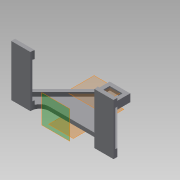
# Autodesk Inventor part: 11_Objektaufnahme
Saved by Autodesk Inventor 2015 (Build 190159000, 159)
## iProperties
Created: 2015-10-26
Part Number: 11_Objektaufnahme
Material: Generisch
Document SubType Name: Modeling
Designer: Bene
Density: 1 g/cm^3
Appearance: Vorgabe
Author: Bene
Autodesk Inventor part; units mm, degrees
ref_plane "YZ Plane" through (0, 0, 0) normal (1, 0, 0) x (0, 1, 0)
ref_plane "XZ Plane" through (0, 0, 0) normal (0, 1, 0) x (-1, 0, 0)
ref_plane "XY Plane" through (0, 0, 0) normal (0, 0, 1) x (1, 0, 0)
ref_plane "Arbeitsebene1" through (0, 0, 0) normal (0, 0, 1) x (1, 0, 0)
ref_plane "Arbeitsebene2" through (0, 0, 0) normal (0, 0, 1) x (1, 0, 0)
ref_plane "Arbeitsebene6" through (0, 0, 5) normal (0, 0, 1) x (1, 0, 0)
sketch "Skizze3" plane through (0, 0, 0) normal (0, 0, 1) x (1, 0, 0)
  line L0 (17.59, -30) -> (0, -30)
  line L1 (0, -30) -> (0, -33)
  line L2 (0, -33) -> (17.59, -33)
  line L3 (17.59, -33) -> (17.59, -30)
  line L4 (-31.8605, -30) -> (48.1395, -30)
  line L5 (48.1395, -30) -> (48.1395, -33)
  line L6 (48.1395, -33) -> (-31.8605, -33)
  line L7 (-31.8605, -33) -> (-31.8605, -30)
  line L8 (-31.8605, -30) -> (48.1395, -33) construction
  line L9 (48.1395, -30) -> (-31.8605, -33) construction
  point P0 (0, 0)
  point P1 (8.1395, -31.5)
  dimension "d9" = 80
  dimension "d10" = 3
  dimension "d11" = 0
  constraints: 20 end point, 2 midpoint, 2 parallel, 1 horizontal, 1 perpendicular
  measures "d9" distance of L5.end L6.end
  measures "d10" distance of L4.end L5.end
  measures "d11" distance between parallel lines of L2 L6
extrude "Extrusion3" add sketch "Skizze3" along normal blind 40
ref_plane "Arbeitsebene4" through (0, -30, 3) normal (0, 1, 0) x (1, 0, 0)
ref_plane "Arbeitsebene5" through (0, -30, 3) normal (0, 1, 0) x (1, 0, 0)
sketch "Skizze5" plane through (0, -30, 3) normal (0, 1, 0) x (1, 0, 0)
  line L0 (-31.8605, 3) -> (48.1395, 3) projected
  line L1 (-31.8605, 3) -> (-31.8605, -37) projected
  line L2 (48.1395, -37) -> (-31.8605, -37) projected
  line L3 (48.1395, 3) -> (48.1395, -37) projected
  line L4 (48.1395, 3) -> (48.1395, -37) projected
  line L5 (-31.8605, -3) -> (48.1395, -3)
  line L6 (48.1395, -3) -> (48.1395, -31)
  line L7 (48.1395, -31) -> (-31.8605, -31)
  line L8 (-31.8605, -31) -> (-31.8605, -3)
  line L9 (-31.8605, -3) -> (48.1395, -31) construction
  line L10 (48.1395, -3) -> (-31.8605, -31) construction
  point P0 (8.1395, -17)
  dimension "d25" = 28
  constraints: 12 end point, 2 midpoint, 2 parallel, 1 horizontal, 1 perpendicular, 1 point on line
  measures "d25" distance of L5.end L6.end
extrude "Extrusion5" cut sketch "Skizze5" against normal blind 1.5 contours L5 L3 L7 L1
sketch "Skizze6" plane through (-31.8605, -30, 0) normal (0, 1, 0) x (1, 0, 0)
  line L0 (0, -6) -> (80, -6) projected
  line L1 (80, 0) -> (80, -6) projected
  line L2 (0, 0) -> (80, 0) projected
  line L3 (0, 0) -> (0, -6) projected
  line L4 (0, -6) -> (80, -6) projected
  line L5 (32, 0) -> (48, 0)
  line L6 (48, 0) -> (48, -6)
  line L7 (48, -6) -> (32, -6)
  line L8 (32, -6) -> (32, 0)
  line L9 (32, 0) -> (48, -6) construction
  line L10 (48, 0) -> (32, -6) construction
  point P0 (40, -3)
  dimension "d26" = 16
  constraints: 12 end point, 2 midpoint, 2 parallel, 1 horizontal, 1 perpendicular, 1 point on line
  measures "d26" distance of L6.end L7.end
ref_plane "Arbeitsebene3" through (-30.5754, 12, -63.8875) normal (0, 1, 0) x (0, 0, 1)
extrude "Extrusion6" add sketch "Skizze6" along normal up to surface (42 mm away) contours L8 L2 L6 L0
chamfer "Fase2" distance 32 angle 45 2 edges at (0.1395, -30, 3) (16.1395, -30, 3)
shell "Wandung1" thickness 3 removed faces 1 at (5.4729, -20.3334, 6)
sketch "Skizze7" plane through (0, -31.5, 3) normal (0, 1, 0) x (1, 0, 0)
  line L0 (48.1395, -3) -> (48.1395, -31) projected
  line L1 (-31.8605, -3) -> (48.1395, -3) projected
  line L2 (-31.8605, -31) -> (-31.8605, -3) projected
  line L3 (48.1395, -31) -> (-31.8605, -31) projected
  line L4 (-16.8605, -4) -> (33.1395, -4)
  line L5 (33.1395, -4) -> (33.1395, -30)
  line L6 (33.1395, -30) -> (-16.8605, -30)
  line L7 (-16.8605, -30) -> (-16.8605, -4)
  line L8 (-16.8605, -4) -> (33.1395, -30) construction
  line L9 (33.1395, -4) -> (-16.8605, -30) construction
  point P0 (0, 3)
  point P1 (8.1395, -17)
  dimension "d28" = 50
  dimension "d29" = 26
  constraints: 12 end point, 2 midpoint, 2 parallel, 1 horizontal, 1 perpendicular
  measures "d28" distance of L5.end L6.end
  measures "d29" distance of L4.end L5.end
extrude "Extrusion7" cut sketch "Skizze7" against normal blind 10 contours L4 L5 L6 L7
sketch "Skizze8" plane through (0, 0, 40) normal (0, 0, 1) x (1, 0, 0)
  line L0 (-31.8605, -33) -> (48.1395, -33) projected
  line L1 (-16.8605, -31.5) -> (-16.8605, -33) projected
  line L2 (48.1395, -30) -> (-31.8605, -30) projected
  line L3 (-31.8605, -30) -> (-31.8605, -33) projected
  line L4 (-31.8605, -33) -> (48.1395, -33) projected
  line L5 (48.1395, -33) -> (48.1395, -30) projected
  line L6 (43.8969, -30) -> (13.1395, 0.7574) projected
  line L7 (13.1395, 0.7574) -> (13.1395, 9) projected
  line L8 (3.1395, 9) -> (13.1395, 9) projected
  line L9 (3.1395, 0.7574) -> (3.1395, 9) projected
  line L10 (3.1395, 0.7574) -> (-27.6178, -30) projected
  line L11 (43.8969, -30) -> (-27.6178, -30) projected
  line L12 (-16.8605, -31.5) -> (-16.8605, -8.6602) construction
  line L13 (-16.8605, -25.5442) -> (7.5954, -1.0883) construction
  line L14 (7.5954, -1.0883) -> (7.5954, 4.5442) construction
  line L15 (7.5954, 4.5442) -> (8.6837, 4.5442) construction
  line L16 (8.6837, 4.5442) -> (8.6837, -1.0883) construction
  line L17 (8.6837, -1.0883) -> (33.1395, -25.5442) construction
  line L18 (33.1395, -25.5442) -> (-16.8605, -25.5442) construction
  line L19 (-16.8605, -33) -> (33.1395, -33)
  line L20 (33.1395, -33) -> (33.1395, -25.5442)
  line L21 (33.1395, -25.5442) -> (-16.8605, -25.5442)
  line L22 (-16.8605, -25.5442) -> (-16.8605, -33)
  point P0 (0, 0)
  point P1 (33.1395, -31.5)
  constraints: 22 end point, 2 parallel, 2 perpendicular, 1 horizontal, 1 point on line, 5 other
extrude "Extrusion8" cut sketch "Skizze8" against normal through all contours L1 L22 L2 L20 L0 | L2 L22 L21 L20
fillet "Rundung1" radius 7 2 edges at (-16.8605, -25.5442, 1.5) (33.1395, -25.5442, 1.5)
